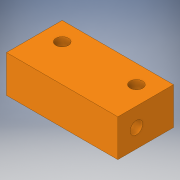
# Autodesk Inventor part: MotorSpacerBlock2
Saved by Autodesk Inventor 2019 (Build 230136000, 136)
## iProperties
Created: 2020-02-28
Part Number: MotorSpacerBlock2
Material: Generic
Document SubType Name: Modeling
Designer: james
Density: 1 g/cm^3
Appearance: Orange
Author: james
Autodesk Inventor part; units mm, degrees
ref_plane "YZ Plane" through (0, 0, 0) normal (1, 0, 0) x (0, 1, 0)
ref_plane "XZ Plane" through (0, 0, 0) normal (0, 1, 0) x (-1, 0, 0)
ref_plane "XY Plane" through (0, 0, 0) normal (0, 0, 1) x (1, 0, 0)
sketch "Sketch1" plane through (0, 0, 0) normal (1, 0, 0) x (0, 1, 0)
  line L0 (7.8254, 10.5896) -> (-4.8746, 10.5896)
  line L1 (-4.8746, 10.5896) -> (-4.8746, -8.4604)
  line L2 (-4.8746, -8.4604) -> (7.8254, -8.4604)
  line L3 (7.8254, -8.4604) -> (7.8254, 10.5896)
  point P0 (0, 0)
  dimension "d0" = 19.05
  dimension "d1" = 12.7
  constraints: 8 end point, 2 parallel, 1 horizontal, 1 perpendicular
  measures "d0" distance of L2.end L0.start
  measures "d1" distance of L0.start L0.end
extrude "Extrusion1" add sketch "Sketch1" along normal blind 38.1
sketch "Sketch2" plane through (38.1, 0, 0) normal (1, 0, 0) x (0, 0, -1)
  line L0 (-10.5896, 7.8254) -> (-10.5896, -4.8746) projected
  line L1 (8.4604, 7.8254) -> (-10.5896, 7.8254) projected
  point P0 (0, 0)
  point P1 (-4.2396, 1.4754)
  dimension "d4" = 6.35
  dimension "d5" = 6.35
  measures "d4" distance from line of L0 point (-4.24, 1.475)
  measures "d5" distance from line of L1 point (-4.24, 1.475)
hole "Hole1" at (38.1, 1.4754, 4.2396) direction (-1, 0, 0) diameter 4.318 end through all
sketch "Sketch3" plane through (0, 7.8254, 10.5896) normal (0, 1, 0) x (1, 0, 0)
  line L0 (38.1, 19.05) -> (38.1, 0) projected
  line L1 (0, 19.05) -> (0, 0) projected
  line L2 (0, 19.05) -> (38.1, 19.05) projected
  point P0 (0, 10.5896)
  point P1 (6.35, 12.7)
  point P2 (31.75, 12.7)
  dimension "d13" = 6.35
  dimension "d14" = 6.35
  dimension "d15" = 6.35
  dimension "d16" = 0
  measures "d13" distance from line of point (31.75, 12.7) L0
  measures "d14" distance from line of L1 point (6.35, 12.7)
  measures "d15" distance from line of L2 point (31.75, 12.7)
  measures "d16" vertical distance of point (31.75, 12.7) point (6.35, 12.7)
hole "Hole2" at (6.35, 7.8254, -2.1104) at (31.75, 7.8254, -2.1104) direction (0, -1, 0) diameter 4.318 end through all
body "Solid1"
